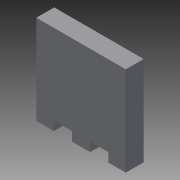
# Autodesk Inventor part: castlegen
Saved by Autodesk Inventor 2014 (Build 180170000, 170)
## iProperties
Created: 2014-07-15
Part Number: castlegen
Material: Generic
Document SubType Name: Modeling
Designer: cruiser
Density: 1 g/cm^3
Appearance: Default
Author: cruiser
Autodesk Inventor part; units mm, degrees
ref_plane "YZ Plane" through (0, 0, 0) normal (1, 0, 0) x (0, 1, 0)
ref_plane "XZ Plane" through (0, 0, 0) normal (0, 1, 0) x (-1, 0, 0)
ref_plane "XY Plane" through (0, 0, 0) normal (0, 0, 1) x (1, 0, 0)
sketch "Sketch1" plane through (0, 0, 0) normal (0, 1, 0) x (-1, 0, 0)
  line L0 (25, -25) -> (-25, -25)
  line L1 (-25, -25) -> (-25, 25)
  line L2 (-25, 25) -> (25, 25)
  line L3 (25, 25) -> (25, -25)
  line L4 (25, -25) -> (-25, 25) construction
  line L5 (-25, -25) -> (25, 25) construction
  point P0 (0, 0)
  dimension "d0" = 50
  dimension "d1" = 50
  constraints: 12 end point, 2 midpoint, 2 parallel, 1 horizontal, 1 perpendicular
  measures "d0" distance of L1.end L2.end
  measures "d1" distance of L0.end L1.end
extrude "Extrusion1" add sketch "Sketch1" along normal blind 10
sketch "Sketch2" plane through (0, 10, 0) normal (0, 1, 0) x (1, 0, 0)
  line L0 (25, 25) -> (-25, 25) projected
  line L1 (0, 0) -> (0, 25)
  line L2 (-5.08, 25) -> (-15.24, 25)
  line L3 (-15.24, 25) -> (-15.24, 19.92)
  line L4 (-15.24, 19.92) -> (-5.08, 19.92)
  line L5 (-5.08, 19.92) -> (-5.08, 25)
  line L6 (5.08, 25) -> (15.24, 25)
  line L7 (15.24, 25) -> (15.24, 19.92)
  line L8 (15.24, 19.92) -> (5.08, 19.92)
  line L9 (5.08, 19.92) -> (5.08, 25)
  dimension "d5" = 5.08
  dimension "d6" = 10.16
  dimension "d7" = 10.16
  dimension "d8" = 10.16
  dimension "d9" = 5.08
  constraints: 18 end point, 4 parallel, 2 horizontal, 2 perpendicular, 2 point on line, 1 coincident, 1 midpoint, 1 other
  measures "d5" distance between parallel lines of L8 L0
  measures "d6" distance between parallel lines of L5 L9
  measures "d7" distance between parallel lines of L7 L9
  measures "d8" distance between parallel lines of L5 L3
  measures "d9" distance of L2.end L3.end
extrude "Extrusion2" cut sketch "Sketch2" against normal up to next
equation "\"d5\" = m2_thickness"
equation "\"d6\" = 2 * m2_thickness"
equation "\"d7\" = 2 * m2_thickness"
equation "\"d8\" = 2 * m2_thickness"
equation "\"d9\" = m2_thickness"
equation "\"m2_thickness\" = 5.08"
body "Solid1"
